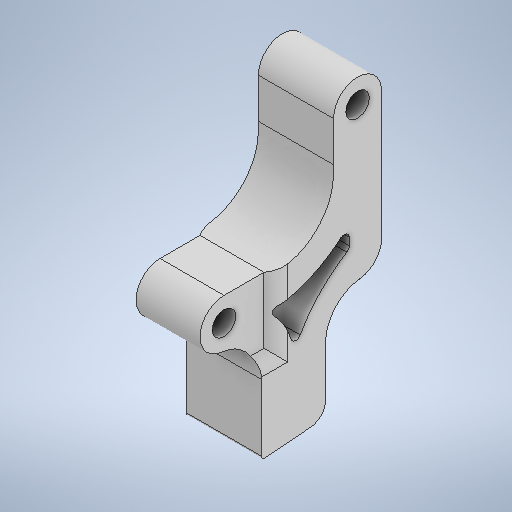
# Autodesk Inventor part: MOGO Mech_oem with mags 2
Saved by Autodesk Inventor 2025.2 (Build 292293000, 293)
## iProperties
Created: 2024-11-22
Part Number: MOGO Mech_oem with mags 2
Material: Generic
Document SubType Name: Modeling
Designer: Juanl
Density: 1 g/cm^3
Appearance: Default
Mass: 11.7203 g
Surface Area: 40.8724 cm^2
Volume: 11.7203 cm^3
Author: Juanl
Autodesk Inventor part; units mm, degrees
ref_plane "YZ Plane" through (0, 0, 0) normal (1, 0, 0) x (0, 1, 0)
ref_plane "XZ Plane" through (0, 0, 0) normal (0, 1, 0) x (-1, 0, 0)
ref_plane "XY Plane" through (0, 0, 0) normal (0, 0, 1) x (1, 0, 0)
sketch "Sketch1" plane through (0, 0, 0) normal (1, 0, 0) x (0, 1, 0)
  line L0 (-12.6683, 12.8416) -> (-12.6683, 0.1416)
  line L1 (-12.6683, 0.1416) -> (-12.6683, -12.5584)
  line L2 (-12.6683, -12.5584) -> (0.0318, -12.5584)
  line L3 (0.0318, -12.5584) -> (12.7318, -12.5584)
  circle A0 centre (-12.6683, 12.8416) radius 2.3241
  circle A1 centre (12.7318, -12.5584) radius 2.3241
  line L4 (-12.6683, 12.8416) -> (-12.6683, -12.5584) construction
  line L5 (-17.4308, 12.8416) -> (-17.4308, -12.5584)
  line L6 (-7.9058, -12.5584) -> (-7.9058, 12.8416)
  arc A2 (-7.9058, 12.8416) -> (-17.4308, 12.8416) centre (-12.6683, 12.8416) ccw
  arc A3 (-17.4308, -12.5584) -> (-7.9058, -12.5584) centre (-12.6683, -12.5584) ccw
  line L7 (12.7318, -12.5584) -> (-12.6683, -12.5584) construction
  line L8 (12.7318, -7.7959) -> (-12.6683, -7.7959)
  line L9 (-12.6683, -17.3209) -> (12.7318, -17.3209)
  arc A4 (12.7318, -17.3209) -> (12.7318, -7.7959) centre (12.7318, -12.5584) ccw
  arc A5 (-12.6683, -7.7959) -> (-12.6683, -17.3209) centre (-12.6683, -12.5584) ccw
  line L10 (-12.6683, 0.1416) -> (-38.0683, 0.1416)
  arc A6 (-7.9058, 4.3417) -> (-7.9058, -4.0585) centre (-12.6683, 0.1416) ccw
  line L11 (-12.6683, 6.4916) -> (-34.8933, 6.4916)
  line L12 (-38.0683, 3.3166) -> (-38.0683, -3.0334)
  line L13 (-34.8933, -6.2084) -> (-12.6683, -6.2084)
  arc A7 (-34.8933, 6.4916) -> (-38.0683, 3.3166) centre (-34.8933, 3.3166) ccw
  arc A8 (-38.0683, -3.0334) -> (-34.8933, -6.2084) centre (-34.8933, -3.0334) ccw
  point P0 (0, 0)
  point P1 (0.0317, -12.5584)
  point P2 (-7.9058, -7.7959)
  point P3 (-17.4308, -6.2084)
  point P4 (-17.4308, 6.4916)
  dimension "d1" = 4.6482
  dimension "d2" = 4.6482
  dimension "d3" = 9.525
  dimension "d7" = 25.4
  dimension "d8" = 12.7
  dimension "d9" = 3.175
  constraints: 32 end point, 16 point on circle, 13 tangent, 9 centre point, 5 point on line, 3 coincident, 3 perpendicular, 2 collinear, 2 parallel, 2 vertical, 1 concentric, 1 equal radius, 1 horizontal, 1 midpoint
  measures "d1" diameter of A0
  measures "d2" diameter of A1
  measures "d3" diameter of A3
  measures "d7" distance of L0.end L10.end
  measures "d8" diameter of A6
  measures "d9" radius of A7
extrude "Extrusion1" add sketch "Sketch1" along normal blind 14.9225
fillet "Fillet1" radius 7.62 1 edges at (7.4613, -17.4308, -6.2084)
fillet "Fillet2" radius 7.62 1 edges at (7.4613, -17.4308, 6.4916)
fillet "Fillet7" radius 12.7 1 edges at (7.4613, -7.9058, -7.7959) curvature continuous yes
sketch "Sketch5" plane through (14.9225, 0, 0) normal (1, 0, 0) x (0, 0, -1)
  arc A0 (-12.8416, -7.9058) -> (-13.3301, -17.4056) centre (-12.8416, -12.6683) ccw projected
  arc A1 (-6.4916, -24.9854) -> (-13.3301, -17.4056) centre (-14.1116, -24.9854) ccw projected
  line L0 (-6.4916, -24.9854) -> (-6.4916, -34.8933) projected
  arc A2 (-6.4916, -34.8933) -> (-3.3166, -38.0683) centre (-3.3166, -34.8933) ccw projected
  line L1 (-3.3166, -38.0683) -> (3.0334, -38.0683) projected
  arc A3 (3.0334, -38.0683) -> (6.2084, -34.8933) centre (3.0334, -34.8933) ccw projected
  line L2 (6.2084, -34.8933) -> (6.2084, -24.9854) projected
  arc A4 (13.0468, -17.4056) -> (6.2084, -24.9854) centre (13.8284, -24.9854) ccw projected
  arc A5 (13.0468, -17.4056) -> (17.3209, -12.6683) centre (12.5584, -12.6683) ccw projected
  line L3 (17.3209, -12.6683) -> (17.3209, 12.7318) projected
  arc A6 (17.3209, 12.7318) -> (7.7959, 12.7318) centre (12.5584, 12.7318) ccw projected
  line L4 (7.7959, 12.7318) -> (7.7959, 4.7942) projected
  line L5 (-4.9041, -7.9058) -> (-12.8416, -7.9058) projected
  circle A7 centre (-12.8416, -12.6683) radius 2.3241 projected
  circle A8 centre (12.5584, 12.7318) radius 2.3241 projected
  line L6 (10.9249, -6.909) -> (10.9249, -11.2735)
  arc A9 (-0.1416, -23.8515) -> (-5.0395, -14.3017) centre (-14.1116, -24.9854) ccw
  line L7 (-5.0395, -14.3017) -> (-4.9041, -14.3017)
  arc A10 (10.9249, -11.2735) -> (-0.1416, -23.8515) centre (24.036, -33.9664) ccw
  arc A11 (-5.0395, -14.3017) -> (10.9249, -6.909) centre (-6.5153, 9.8191) ccw
  point P0 (0, 0)
  constraints: 6 point on circle, 4 end point, 3 centre point, 2 other
extrude "Extrusion4" cut sketch "Sketch5" against normal blind 25.4 contours L6 A10 A9 A11
fillet "Fillet8" radius 1.016 1 edges at (7.4613, -14.3017, 5.0395)
fillet "Fillet9" radius 1.016 2 edges at (7.4613, -23.8515, 0.1416) (7.4613, -6.909, -10.9249)
fillet "Fillet10" radius 1.016 1 edges at (7.4613, -11.2735, -10.9249)
sketch "Sketch6" plane through (14.9225, 0, 0) normal (1, 0, 0) x (0, 0, -1)
  arc A0 (-6.4916, -34.8933) -> (-3.3166, -38.0683) centre (-3.3166, -34.8933) ccw projected
  line L0 (-6.4916, -34.8933) -> (-6.4916, -38.0683)
  line L1 (-6.4916, -38.0683) -> (-6.4916, -38.862)
  line L2 (-3.3166, -38.0683) -> (3.0334, -38.0683) projected
  arc A1 (3.0334, -38.0683) -> (6.2084, -34.8933) centre (3.0334, -34.8933) ccw projected
  line L3 (-6.4916, -38.862) -> (3.0334, -38.0683)
  point P0 (0, 0)
  dimension "d26" = 0.7937
  constraints: 6 end point, 1 point on line, 1 tangent, 1 vertical
  measures "d26" distance of L0.end L1.end
extrude "Extrusion5" add sketch "Sketch6" against normal blind 14.9225
fillet "Fillet11" radius 0.635 1 edges at (7.4613, -38.862, 6.4916)
sketch "Sketch7" plane through (0, -38.0683, -3.0334) normal (0, -0.9965458, -0.0830455) x (1, 0, 0)
  line L0 (0, 0) -> (14.9225, 0) projected
  line L1 (0, 2.2874) -> (0, 0.4514) projected
  line L2 (0, 0) -> (0, 2.2874)
  line L3 (0, 2.2874) -> (2.4511, 2.2874)
  line L4 (2.8321, 2.2874) -> (12.0269, 2.2874)
  line L5 (12.4079, 2.6684) -> (12.4079, 6.834)
  line L6 (12.0269, 7.215) -> (2.8321, 7.215)
  line L7 (2.4511, 6.834) -> (2.4511, 2.6684)
  line L8 (14.9225, 8.8679) -> (14.9225, 0) projected
  arc A0 (12.4079, 6.834) -> (12.0269, 7.215) centre (12.0269, 6.834) ccw
  arc A1 (2.4511, 2.6684) -> (2.8321, 2.2874) centre (2.8321, 2.6684) ccw
  arc A2 (12.0269, 2.2874) -> (12.4079, 2.6684) centre (12.0269, 2.6684) ccw
  arc A3 (2.8321, 7.215) -> (2.4511, 6.834) centre (2.8321, 6.834) ccw
  point P0 (0, -0.1385)
  point P1 (12.4079, 7.215)
  point P2 (12.4079, 2.2874)
  point P3 (2.4511, 7.215)
  dimension "d30" = 4.9276
  dimension "d31" = 9.9568
  dimension "d32" = 2.5146
  dimension "d58" = 0.381
  dimension "d59" = 0.381
  constraints: 12 end point, 8 point on circle, 8 point on line, 8 tangent, 4 centre point, 2 equal radius, 2 parallel, 2 perpendicular, 1 collinear, 1 horizontal
  measures "d30" distance of point (12.408, 2.287) point (12.408, 7.215)
  measures "d31" distance of point (12.408, 7.215) point (2.451, 7.215)
  measures "d32" distance between parallel lines of L8 L5
  measures "d58" radius of A0
  measures "d59" radius of A1
extrude "Extrusion6" cut sketch "Sketch7" against normal blind 1.9304
sketch "Sketch12" plane through (14.9225, 0, 0) normal (1, 0, 0) x (0, 0, -1)
  arc A0 (-12.8416, -7.9058) -> (-13.3301, -17.4056) centre (-12.8416, -12.6683) ccw projected
  line L0 (-12.8416, -7.9058) -> (-7.6346, -7.9058)
  line L1 (-4.9041, -7.9058) -> (-12.8416, -7.9058) projected
  line L2 (-7.6346, -7.9058) -> (-7.6346, -20.9714)
  arc A1 (-6.4916, -24.9854) -> (-13.3301, -17.4056) centre (-14.1116, -24.9854) ccw projected
  arc A2 (-12.8416, -7.9058) -> (-13.3301, -17.4056) centre (-12.8416, -12.6683) ccw
  arc A3 (-7.6346, -20.9714) -> (-13.3301, -17.4056) centre (-14.1116, -24.9854) ccw
  line L3 (-6.4916, -20.9714) -> (-6.4916, -7.9058)
  line L4 (-7.6346, -7.9058) -> (-6.4916, -7.9058)
  line L5 (-4.9041, -7.9058) -> (-4.9041, -20.9714)
  line L6 (-7.6346, -20.9714) -> (-4.9041, -20.9714)
  point P0 (0, 0)
  dimension "d48" = 5.207
  constraints: 12 end point, 5 point on circle, 3 perpendicular, 3 point on line, 2 centre point, 2 tangent, 1 collinear, 1 concentric, 1 vertical
  measures "d48" distance of L0.start L0.end
extrude "Extrusion10" cut sketch "Sketch12" against normal blind 1.1112
sketch "Sketch13" plane through (0, 0, 0) normal (-1, 0, 0) x (0, 0, 1)
  line L0 (4.9041, -7.9058) -> (12.8416, -7.9058) projected
  line L1 (12.8416, -7.9058) -> (7.6346, -7.9058)
  line L2 (7.6346, -7.9058) -> (7.6346, -20.9714)
  arc A0 (13.3301, -17.4056) -> (6.4916, -24.9854) centre (14.1116, -24.9854) ccw projected
  arc A1 (13.3301, -17.4056) -> (12.8416, -7.9058) centre (12.8416, -12.6683) ccw projected
  arc A2 (13.3301, -17.4056) -> (12.8416, -7.9058) centre (12.8416, -12.6683) ccw
  arc A3 (13.3301, -17.4056) -> (7.6346, -20.9714) centre (14.1116, -24.9854) ccw
  line L3 (7.6346, -7.9058) -> (6.3614, -7.9058)
  line L4 (6.4916, -24.9854) -> (6.4916, -38.1719) projected
  line L5 (6.4916, -20.9714) -> (6.4916, -7.9058)
  line L6 (6.4916, -7.9058) -> (7.6346, -7.9058)
  line L7 (4.9041, -7.9058) -> (4.9041, -20.9714) projected
  line L8 (4.9041, -7.9058) -> (4.9041, -20.9714)
  line L9 (4.9041, -20.9714) -> (7.6346, -20.9714)
  point P0 (0, 0)
  dimension "d51" = 5.207
  constraints: 14 end point, 5 point on circle, 3 point on line, 2 centre point, 2 concentric, 2 perpendicular, 2 vertical
  measures "d51" distance of L0.end L1.end
extrude "Extrusion11" cut sketch "Sketch13" against normal blind 1.1112
fillet "Fillet17" radius 6.35 2 edges at (14.9225, -14.4386, 4.9041) (14.9225, -20.9714, 6.2694)
fillet "Fillet18" radius 6.35 2 edges at (0, -14.4386, 4.9041) (0, -20.9714, 6.2694)
body "Solid1"
